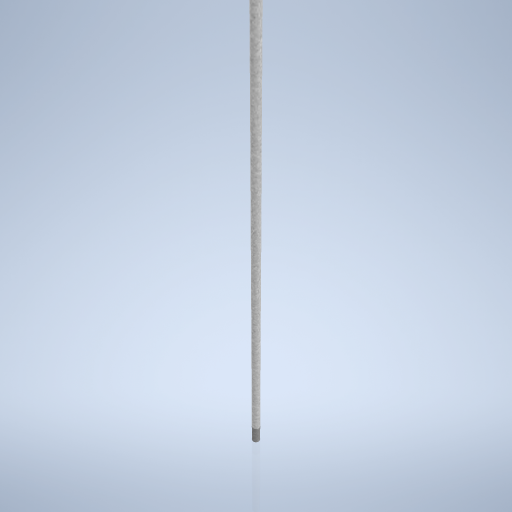
# Autodesk Inventor part: welle
Saved by Autodesk Inventor 2024.2 (Build 282272000, 272)
## iProperties
Created: 2024-05-05
Part Number: welle
Material: Glasfaserbeton
Document SubType Name: Modeling
Designer: Fabri
Density: 1.7 g/cm^3
Appearance: Flach - Poliert Grau
Author: Fabri
Autodesk Inventor part; units mm, degrees
ref_plane "YZ Plane" through (0, 0, 0) normal (1, 0, 0) x (0, 1, 0)
ref_plane "XZ Plane" through (0, 0, 0) normal (0, 1, 0) x (-1, 0, 0)
ref_plane "XY Plane" through (0, 0, 0) normal (0, 0, 1) x (1, 0, 0)
sketch "Skizze1" plane through (0, 0, 0) normal (0, 1, 0) x (-1, 0, 0)
  line L0 (0, 0) -> (3, 0)
  line L1 (3, 0) -> (3, -10.5)
  line L2 (3, -10.5) -> (3.75, -10.5)
  line L3 (3.75, -10.5) -> (3.75, -408.5)
  line L4 (3.75, -408.5) -> (0, -408.5)
  line L5 (0, -408.5) -> (0, 0)
  point P0 (1.5, 0)
  dimension "d0" = 10.5
  dimension "d1" = 398
  dimension "d3" = 6
  dimension "d4" = 7.5
  constraints: 12 end point, 4 perpendicular, 1 midpoint, 1 parallel, 1 vertical
  measures "d0" distance from line of L2 point (1.5, 0)
  measures "d1" distance between parallel lines of L4 L2
  measures "d3" diameter of L1 L5
  measures "d4" diameter of L3 L5
revolve "Umdrehung1" add sketch "Skizze1" angle 360 about axis through (0, 0, -408.5) along (0, 0, 1)
thread "Gewinde1" size "M6x1" class "6g" standard "ISO Metric profile" full length
thread "Gewinde2" size "M8x1.25" class "6g" standard "ISO Metric profile" length 18
